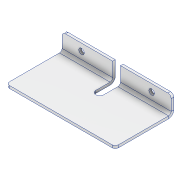
# Autodesk Inventor part: backing plate lidar
Saved by Autodesk Inventor 2020.3 (Build 243373000, 373)
## iProperties
Created: 2020-10-19
Part Number: backing plate lidar
Material: Aluminum 6061
Document SubType Name: Sheet Metal
Designer: Svend
Density: 2.7 g/cm^3
Sheet Metal Rule: Default_mm
Appearance: Aluminum - Flat
Author: Svend
Autodesk Inventor part; units mm, degrees
ref_plane "YZ Plane" through (0, 0, 0) normal (1, 0, 0) x (0, 1, 0)
ref_plane "XZ Plane" through (0, 0, 0) normal (0, 1, 0) x (-1, 0, 0)
ref_plane "XY Plane" through (0, 0, 0) normal (0, 0, 1) x (1, 0, 0)
sketch "Sketch1" plane through (0, 0, 0) normal (0, 0, 1) x (1, 0, 0)
  line L0 (0, 0) -> (84, 0)
  line L1 (84, 0) -> (84, 15)
  line L2 (84, 15) -> (0, 15)
  line L3 (0, 15) -> (0, 0)
  dimension "d0" = 84
  dimension "d1" = 15
  measures "d0" distance of L2.end L1.end
  measures "d1" distance of L1.end L0.end
extrude "Plate1" add sketch "Sketch1" along normal blind 2
sketch "Sketch2" plane through (84, 2, 0) normal (0, -1, 0) x (1, 0, 0)
  line L0 (-84, 0) -> (0, 0)
  line L1 (0, 0) -> (0, 45)
  line L2 (0, 45) -> (-84, 45)
  line L3 (-84, 45) -> (-84, 0)
  constraints: 6 end point, 1 horizontal, 1 perpendicular, 1 vertical
edge flange "Flange1" height 45 angle 90 thickness 2 bend radius 2 thickness toward (0, -1, 0) relief straight relief width 2 relief depth 1 edges at (42, 0, 2) wall of the first edge with corners at (0, 2, 0) (84, 2, 0) (84, 2, 45) (0, 2, 45)
bend "Bend1"
corner "Corner1"
sketch "Sketch3" plane through (0, 0, 0) normal (0, 0, -1) x (-1, 0, 0)
  line L0 (-84, 4) -> (0, 4) projected
  line L1 (0, 15) -> (0, 4) projected
  line L2 (-84, 15) -> (0, 15) projected
  line L3 (-84, 4) -> (-84, 15) projected
  circle A0 centre (-15, 9.5) radius 2.1
  circle A1 centre (-69, 9.5) radius 2.1
  point P0 (0, 0)
  point P1 (-84, 9.5)
  dimension "d13" = 15
  dimension "d14" = 15
  dimension "d15" = 4.2
  constraints: 2 centre point, 2 horizontal alignment, 1 equal radius, 1 midpoint
  measures "d13" distance from line of L3 A1.centre
  measures "d14" distance from line of L1 A0.centre
  measures "d15" diameter of A0
extrude "Cut1" cut sketch "Sketch3" against normal blind 2 contours A0 | A1
fillet "Corner Round1" radius 2.5 4 edges at (84, 15, 1) (0, 15, 1) (0, 1, 45) (84, 1, 45)
sketch "Sketch5" plane through (0, 0, 4) normal (0, -1, 0) x (1, 0, 0)
  arc A0 (84, 38.5) -> (81.5, 41) centre (81.5, 38.5) ccw projected
  line L0 (2.5, 41) -> (81.5, 41) projected
  arc A1 (2.5, 41) -> (0, 38.5) centre (2.5, 38.5) ccw projected
  line L1 (0, 0) -> (0, 38.5) projected
  line L2 (0, 0) -> (84, 0) projected
  line L3 (84, 38.5) -> (84, 0) projected
  line L4 (84, -4) -> (84, 0) projected
  line L5 (0, 0) -> (0, -4) projected
  line L6 (84, -4) -> (0, -4) projected
  line L7 (81.5, -4) -> (2.5, -4) projected
  line L8 (45, 11) -> (39, 11)
  line L9 (39, 11) -> (39, -4)
  line L10 (39, -4) -> (45, -4)
  line L11 (45, -4) -> (45, 11)
  line L12 (45, 11) -> (39, -4) construction
  line L13 (39, 11) -> (45, -4) construction
  circle A2 centre (42, 11) radius 3
  point P0 (42, 3.5)
  point P1 (42, -4)
  dimension "d24" = 6
  dimension "d25" = 15
  constraints: 12 end point, 4 midpoint, 2 parallel, 1 horizontal, 1 horizontal alignment, 1 perpendicular, 1 point on line, 1 vertical alignment, 2 other
  measures "d24" distance between parallel lines of L11 L9
  measures "d25" distance between parallel lines of L7 L8
extrude "Cut3" cut sketch "Sketch5" against normal through all contours L11 L6 L9 L2 | L2 L9 A2 L11 | A2 L8 | L8 A2
equation "\"d14\" = d13"
equation "\"d16\" = Thickness"
equation "\"d26\" = Thickness"
equation "\"d2\" = Thickness"
equation "\"d3\" = BendReliefWidth"
equation "\"d4\" = BendReliefDepth"
equation "\"d5\" = MinimumRemnant"
equation "\"d6\" = TransitionRadius"
equation "\"d9\" = BendRadius"
equation "\"d10\" = CornerReliefSize"
equation "\"d11\" = GapSize"
equation "\"d12\" = JacobiRadiusSize"
equation "\"BendRadius\" = Thickness"
equation "\"BendReliefWidth\" = Thickness"
equation "\"BendReliefDepth\" = 0.5 * Thickness"
equation "\"CornerReliefSize\" = 4 * Thickness"
equation "\"MinimumRemnant\" = 2 * Thickness"
equation "\"TransitionRadius\" = BendRadius"
equation "\"JacobiRadiusSize\" = BendRadius"
equation "\"GapSize\" = Thickness"
equation "\"Thickness\" = 2"
body "Solid1"
